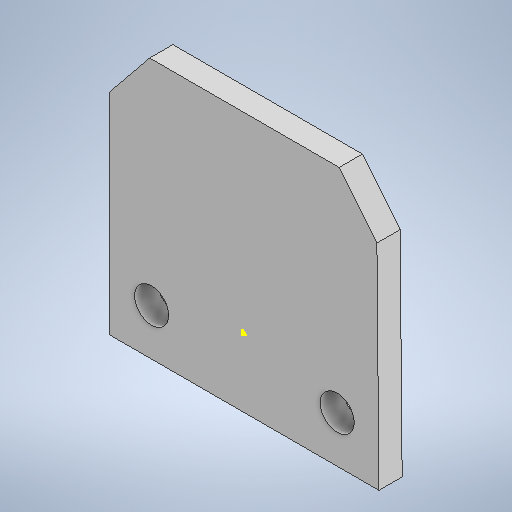
# Autodesk Inventor part: Hook
Saved by Autodesk Inventor 2025.1 (Build 291241020, 241B)
## iProperties
Created: 2024-11-21
Part Number: Hook
Material: Generic
Document SubType Name: Modeling
Designer: AtuStem
Density: 1 g/cm^3
Appearance: Default
Author: AtuStem
Autodesk Inventor part; units mm, degrees
ref_plane "YZ Plane" through (0, 0, 0) normal (1, 0, 0) x (0, 1, 0)
ref_plane "XZ Plane" through (0, 0, 0) normal (0, 1, 0) x (-1, 0, 0)
ref_plane "XY Plane" through (0, 0, 0) normal (0, 0, 1) x (1, 0, 0)
sketch "Sketch1" plane through (0, 0, 0) normal (0, 0, 1) x (1, 0, 0)
  line L0 (-22.225, 9.525) -> (22.225, 9.525)
  line L1 (22.225, 9.525) -> (22.225, -9.525)
  line L2 (22.225, -9.525) -> (-22.225, -9.525)
  line L3 (-22.225, -9.525) -> (-22.225, 9.525)
  line L4 (-22.225, 9.525) -> (22.225, -9.525) construction
  line L5 (22.225, 9.525) -> (-22.225, -9.525) construction
  point P0 (0, 0)
  dimension "d0" = 44.45
  dimension "d18" = 19.05
  constraints: 12 end point, 2 midpoint, 2 parallel, 1 horizontal, 1 perpendicular
  measures "d0" distance of L1.end L2.end
  measures "d18" distance of L2.end L0.start
extrude "Extrusion1" add sketch "Sketch1" along normal blind 3.175
sketch "Sketch2" plane through (22.225, -9.525, 0) normal (1, 0, 0) x (0, 0, -1)
  line L0 (0, 0) -> (0, 19.05) projected
  line L1 (-3.175, 19.05) -> (0, 19.05)
  line L2 (0, 19.05) -> (0, 48.26)
  line L3 (0, 48.26) -> (-3.175, 48.26)
  line L4 (-3.175, 48.26) -> (-3.175, 19.05)
  line L5 (-3.175, 19.05) -> (0, 19.05)
  point P0 (0, 9.525)
  dimension "d27" = 29.21
  constraints: 10 end point, 4 perpendicular, 1 vertical
  measures "d27" distance of L0.end L2.end
extrude "Extrusion2" add sketch "Sketch2" against normal blind 44.45 fills toward (-0.05, 33.655) open curves L2 L3 L4
sketch "Sketch5" plane through (0, 0, 3.175) normal (0, 0, 1) x (1, 0, 0)
  line L0 (-22.225, -9.525) -> (22.225, -9.525) projected
  line L1 (-22.225, -9.525) -> (-22.225, -3.175)
  line L2 (-22.225, 9.525) -> (-22.225, -9.525) projected
  line L3 (-22.225, -3.175) -> (22.225, -3.175)
  line L4 (22.225, -3.175) -> (22.225, -9.525)
  line L5 (-22.225, -3.175) -> (0, -3.175)
  line L6 (-11.1125, -3.175) -> (14.2875, -3.175)
  line L7 (-22.225, -3.175) -> (-12.7, -3.175)
  line L8 (-12.7, -3.175) -> (12.7, -3.175)
  line L9 (12.7, -3.175) -> (22.225, -3.175)
  circle A0 centre (-12.7, -3.175) radius 2.3241
  circle A1 centre (12.7, -3.175) radius 2.3241
  point P0 (0, 0)
  dimension "d11" = 6.35
  dimension "d23" = 9.525
  dimension "d24" = 25.4
  dimension "d25" = 4.6482
  dimension "d26" = 4.6482
  constraints: 16 end point, 4 point on line, 2 centre point, 2 coincident, 2 midpoint, 1 collinear, 1 horizontal, 1 perpendicular
  measures "d11" distance of L0.start L1.end
  measures "d23" distance of L1.end L7.end
  measures "d24" distance of L7.end L8.end
  measures "d25" diameter of A0
  measures "d26" diameter of A1
extrude "Extrusion4" cut sketch "Sketch5" against normal blind 50.8 contours A0 L3 | L3 A0 | A1 L3 | L3 A1
sketch "Sketch6" plane through (0, 0, 3.175) normal (0, 0, 1) x (1, 0, 0)
  point P0 (0, 0)
sketch "Sketch7" plane through (0, 0, 3.175) normal (0, 0, 1) x (1, 0, 0)
  line L0 (-22.225, -9.525) -> (-22.225, 38.735) projected
  line L1 (-22.225, 14.605) -> (-2.6849, 38.735)
  line L2 (22.225, 38.735) -> (-22.225, 38.735) projected
  line L3 (22.225, -9.525) -> (22.225, 38.735) projected
  line L4 (22.225, 14.605) -> (2.6849, 38.735)
  line L5 (-2.6849, 38.735) -> (-22.225, 38.735)
  line L6 (-22.225, 14.605) -> (-22.225, 14.605)
  line L7 (-22.225, 38.735) -> (-22.225, 14.605)
  line L8 (22.225, 14.605) -> (22.225, 38.735)
  line L9 (22.225, 38.735) -> (2.6849, 38.735)
  point P0 (0, 0)
  dimension "d29" = 39
  dimension "d30" = 39
  constraints: 14 end point, 3 collinear, 3 point on line, 2 midpoint, 1 perpendicular
  measures "d29" angle of L0 L1
  measures "d30" angle of L3 L4
extrude "Extrusion5" cut sketch "Sketch7" along normal through all both and the other way through all
sketch "Sketch8" plane through (0, 0, 3.175) normal (0, 0, 1) x (1, 0, 0)
  line L0 (-22.225, -9.525) -> (22.225, -9.525) projected
  line L1 (0, -9.525) -> (0, 26.035)
  line L2 (0, 26.035) -> (-19.9542, 26.035)
  line L3 (-19.9542, 26.035) -> (-19.9542, 44.6451)
  line L4 (-19.9542, 44.6451) -> (20.0631, 44.6451)
  line L5 (20.0631, 44.6451) -> (20.0631, 26.035)
  line L6 (20.0631, 26.035) -> (0, 26.035)
  point P0 (0, 0)
  dimension "d33" = 35.56
  constraints: 12 end point, 4 perpendicular, 1 horizontal, 1 midpoint, 1 point on line, 1 vertical
  measures "d33" distance of L1.start L1.end
extrude "Extrusion6" cut sketch "Sketch8" against normal through all
sketch "Sketch9" plane through (0, 0, 3.175) normal (0, 0, 1) x (1, 0, 0)
  line L0 (-22.225, 14.605) -> (-22.225, -9.525) projected
  line L1 (-22.225, -9.525) -> (-18.415, -9.525)
  line L2 (-22.225, -9.525) -> (22.225, -9.525) projected
  line L3 (-18.415, -9.525) -> (-18.415, 28.0606)
  line L4 (-18.415, 28.0606) -> (-22.225, 28.0606)
  line L5 (-22.225, 28.0606) -> (-22.225, -9.525)
  line L6 (22.225, -9.525) -> (18.415, -9.525)
  line L7 (18.415, -9.525) -> (18.0562, 28.0606)
  line L8 (18.0562, 28.0606) -> (22.225, 28.0606)
  line L9 (22.225, 28.0606) -> (22.225, -9.525)
  point P0 (0, 0)
  dimension "d36" = 3.81
  dimension "d37" = 3.81
  constraints: 16 end point, 4 perpendicular, 4 point on line
  measures "d36" distance of L0.end L1.end
  measures "d37" distance of L2.end L6.end
extrude "Extrusion7" cut sketch "Sketch9" against normal blind 25.4
body "Solid1"
